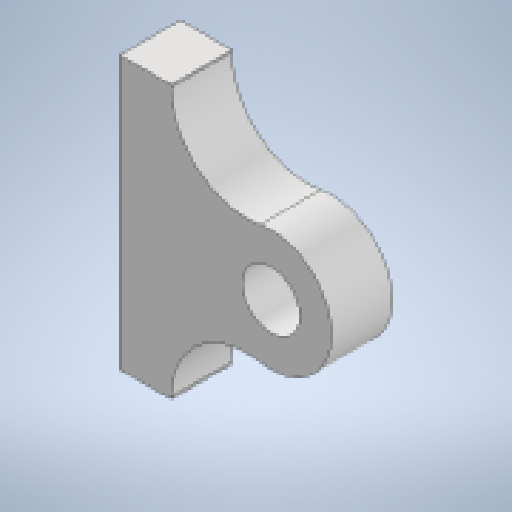
# Autodesk Inventor part: Bracket
Saved by Autodesk Inventor 2024 (Build 280153000, 153)
## iProperties
Created: 2024-01-04
Part Number: Bracket
Material: Generic
Document SubType Name: Modeling
Designer: student
Density: 1 g/cm^3
Appearance: Default
Author: student
Autodesk Inventor part; units mm, degrees
ref_plane "YZ Plane" through (0, 0, 0) normal (1, 0, 0) x (0, 1, 0)
ref_plane "XZ Plane" through (0, 0, 0) normal (0, 1, 0) x (-1, 0, 0)
ref_plane "XY Plane" through (0, 0, 0) normal (0, 0, 1) x (1, 0, 0)
sketch "Sketch1" plane through (0, 0, 0) normal (0, 0, 1) x (1, 0, 0)
  circle A0 centre (0, 0) radius 6 projected
  circle A1 centre (0, 0) radius 12.7
  line L0 (-31.75, -28.575) -> (-31.75, 42.3507)
  line L1 (0, 0) -> (0, 6)
  line L2 (-31.75, -28.575) -> (-20.955, -28.575)
  line L3 (-20.955, 28.575) -> (-31.75, 28.575)
  line L4 (-31.75, 28.575) -> (-31.75, -28.575)
  line L5 (0, 0) -> (6, 0)
  arc A2 (-2.2578, -12.4977) -> (-20.955, -28.1198) centre (-5.08, -28.1198) ccw
  arc A3 (-20.955, 28.1198) -> (-2.2578, 12.4977) centre (-5.08, 28.1198) ccw
  line L6 (-20.955, -28.575) -> (-20.955, -28.1198)
  line L7 (-20.955, 28.1198) -> (-20.955, 28.575)
  point P0 (0, 0)
  dimension "d0" = 31.75
  dimension "d1" = 25.4
  dimension "d2" = 57.15
  dimension "d3" = 10.795
  dimension "d4" = 31.75
  dimension "d5" = 31.75
  constraints: 16 end point, 8 point on circle, 6 tangent, 4 parallel, 3 centre point, 2 horizontal, 2 perpendicular, 1 vertical, 1 other
  measures "d0" distance between parallel lines of L1 L0
  measures "d1" diameter of A1
  measures "d2" distance of L2.end L3.start
  measures "d3" distance of L0.start L2.end
  measures "d4" diameter of A2
  measures "d5" diameter of A3
extrude "Extrusion1" add sketch "Sketch1" along normal blind 12.7
sketch "Sketch2" plane through (-20.955, -28.575, 0) normal (1, 0, 0) x (0, 0, -1)
  circle A0 centre (-6.35, 6.35) radius 4.1275
  circle A1 centre (-6.35, 50.8) radius 4.1275
  line L0 (0, 28.575) -> (-16.7111, 28.575)
  line L1 (0, 0) -> (-12.7, 0) projected
  line L2 (0, 57.15) -> (-12.7, 57.15) projected
  point P0 (-6.35, 0)
  dimension "d8" = 8.255
  dimension "d9" = 6.35
  dimension "d10" = 6.35
  constraints: 2 centre point, 2 end point, 2 vertical alignment, 1 horizontal, 1 midpoint, 1 other
  measures "d8" diameter of A0
  measures "d9" distance from line of L1 A0.centre
  measures "d10" distance from line of L2 A1.centre
extrude "Extrusion2" cut sketch "Sketch2" along normal through all
sketch "Sketch3" plane through (-20.955, -22.225, 6.35) normal (1, 0, 0) x (0, 0, -1)
  circle A0 centre (0, 0) radius 4.1275 projected
  circle A1 centre (0, 44.45) radius 4.1275 projected
  point P0 (6.35, 22.225)
extrude "Extrusion3" cut sketch "Sketch3" against normal blind 6.35
sketch "Sketch4" plane through (-27.305, -22.225, 6.35) normal (1, 0, 0) x (0, 0, -1)
  circle A0 centre (0, 0) radius 4.1275 projected
  circle A1 centre (0, 0) radius 2.54
  circle A2 centre (0, 44.45) radius 4.1275 projected
  circle A3 centre (0, 44.45) radius 4.1275 projected
  circle A4 centre (0, 44.45) radius 2.54
  point P0 (6.35, 22.225)
  dimension "d15" = 5.08
  dimension "d16" = 5.08
  constraints: 2 centre point, 2 coincident
  measures "d15" diameter of A1
  measures "d16" diameter of A4
extrude "Extrusion4" cut sketch "Sketch4" against normal through all contours A1 | A4
fillet "Fillet1" radius 6.35 4 edges at (-26.3525, -28.575, 12.7) (-26.3525, -28.575, 0) (-26.3525, 28.575, 12.7) (-26.3525, 28.575, 0)
sketch "Sketch5" plane through (0, 0, 12.7) normal (0, 0, 1) x (1, 0, 0)
  circle A0 centre (0, 0) radius 9.525
  dimension "d20" = 19.05
  constraints: 1 centre point, 1 coincident
  measures "d20" diameter of A0
extrude "Extrusion5" cut sketch "Sketch5" against normal blind 6.35
body "Solid1"
